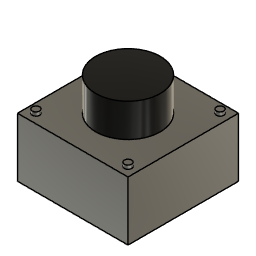
NO MOMENTARY SWITCH v2 (Autodesk Fusion 360 design; units mm, degrees)
Autodesk Fusion 360 part; units mm, degrees
sketch "Sketch1" plane through (0, 0, 0) normal (0, 0, 1) x (1, 0, 0)
  line L0 (-3, 3) -> (3, 3)
  line L1 (3, 3) -> (3, -3)
  line L2 (3, -3) -> (-3, -3)
  line L3 (-3, -3) -> (-3, 3)
  dimension "d1" = 6
  dimension "d2" = 6
  dimension "d3" = 3
  dimension "d4" = 3
  constraint horizontal L0
  constraint vertical L1
  constraint horizontal L2
  constraint vertical L3
  measures "d1" distance of L0.start L0.end
  measures "d2" distance of L0.start L2.end
  measures "d3" distance of origin L1
  measures "d4" distance of origin L2
extrude "Extrude1" add sketch "Sketch1" along normal blind 2.5 makes body 1
sketch "Sketch2" plane through (0, 0, 2.5) normal (0, 0, 1) x (-1, 0, 0)
  line L0 (3, 3) -> (-3, 3)
  line L1 (-3, 3) -> (-3, -3)
  line L2 (-3, -3) -> (3, -3)
  line L3 (3, -3) -> (3, 3)
  circle A0 centre (0, 0) radius 1.75
  circle A1 centre (2.5, -2.5) radius 0.2
  circle A2 centre (2.5, 2.5) radius 0.2
  circle A3 centre (-2.5, 2.5) radius 0.2
  circle A4 centre (-2.5, -2.5) radius 0.2
  dimension "d7" = 3.5
  dimension "d8" = 0.4
  dimension "d9" = 0.4
  dimension "d10" = 0.4
  dimension "d11" = 0.4
  constraint coincident A0.centre origin
  measures "d7" diameter of A0
  measures "d8" diameter of A1
  measures "d9" diameter of A2
  measures "d10" diameter of A3
  measures "d11" diameter of A4
extrude "Extrude2" add sketch "Sketch2" along normal blind 0.4 contours A1 | A2 | A3 | A4 bodies 1
extrude "Extrude3" add sketch "Sketch2" along normal blind 1.8 contours A0 bodies 1
extrude "Extrude4" add 1 faces at (-1, -1, 0) along direction (0, 0, -1) blind 0.7 on bodies 1 bodies 1
extrude "Extrude5" cut 4 faces at (2.5659, -2.6006, 2.9) (2.5659, 2.3994, 2.9) (-2.4341, 2.3994, 2.9) (-2.4341, -2.6006, 2.9) along direction (0, 0, -1) blind 0.2 on bodies 1 bodies 1
delete_face "DeleteFace1" 2 faces at (0.482, -0.4649, 4.3) (-1.7478, 0.0872, 3.7) on bodies 1
extrude "Extrude6" add sketch "Sketch2" along normal blind 1.8 separate body contours A0 makes body 2
named bodies: "Switch Body", "Button"
